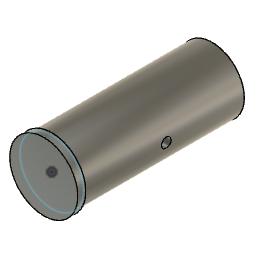
Small wrapped collar design _24 v3 (Autodesk Fusion 360 design; units mm, degrees)
Autodesk Fusion 360 part; units mm, degrees
sketch "Sketch2" plane through (0, 0, 0) normal (0, 0, 1) x (1, 0, 0)
  line L0 (0, 25.4) -> (10.16, 25.4)
  line L1 (0, 25.4) -> (0, 76.2)
  line L2 (10.16, 25.4) -> (10.16, 76.2)
  line L3 (10.16, 76.2) -> (0, 76.2)
  dimension "d47" = 10.16
  dimension "d48" = 50.8
  dimension "d49" = 50.8
  constraint horizontal L0
  constraint perpendicular L0 L1
  constraint perpendicular L0 L2
  measures "d47" distance of L0.start L0.end
  measures "d48" distance of L0.start L1.end
  measures "d49" distance of L0.end L2.end
revolve "Revolve1" add sketch "Sketch2" angle 360 about axis through (0, 25.4, 0) along (0, 1, 0) makes body 1
sketch "Sketch3" plane through (0, 76.2, 0) normal (0, 1, 0) x (-1, 0, 0)
  circle A0 centre (0, 0) radius 10.16
  circle A1 centre (0, 0) radius 5.08
  dimension "d6" = 10.16
  constraint coincident A0.centre A1.centre
  measures "d6" diameter of A1
sketch "Sketch7" plane through (0, 0, 0) normal (0, 0, 1) x (1, 0, 0)
  circle A0 through (2.5427, 49.9294, -10.5604) (-1.2073, 52.0944, -10.5604) (-1.2073, 47.7643, -10.5604)
  dimension "d15" = 5
sketch "Sketch8" plane through (0, 76.2, 0) normal (0, 1, 0) x (-1, 0, 0)
  circle A0 centre (0, 0) radius 10.16
  circle A1 centre (0, 0) radius 6.35
  dimension "d29" = 12.7
  constraint concentric A0 A1
  measures "d29" diameter of A1
hole "Hole4" at (-0.0344, 76.2, -0.1321) direction (0, -1, 0) diameter 15.3924 depth 50.8 tip angle 180 bodies 1
thread "Thread2" "ANSI Unified Screw Threads 0.6875 11/16-12 UN 2B" major diameter 17.4625 minor diameter 15.3924 pitch 2.1167 angle 60 resizes the face on face at (0.7319, 59.2667, 7.5258) on bodies 1
extrude "Extrude5" add sketch "Sketch3" against normal blind 50.8 separate body contours A1 makes body 2
hole "Hole5" at (-10.16, 51.5126, 0) direction (1, 0, 0) diameter 2.9972 depth 50.292 tip angle 118 bodies 1
move_face "OffsetFaces1" offset -38.1 1 faces at (1.2838, 76.2, 0.6601) on bodies 2
sketch "Sketch9" plane through (0, 25.4, 0) normal (0, -1, 0) x (1, 0, 0)
  circle A0 centre (0, 0) radius 5.08
  circle A1 centre (0, 0) radius 10.0907
  constraint coincident A0.centre A1.centre
sketch "Sketch10" plane through (0, 0, 0) normal (0, 1, 0) x (1, 0, 0)
  circle A0 centre (0, 0) radius 10.7615
  constraint coincident A0.centre origin
extrude "Extrude6" add sketch "Sketch10" along normal blind 2.54 separate body makes body 3
move_body "Move1" bodies 3 to x (1, 0, 0) y (0, 1, 0) z (0, 0, 1) at (0, 22.86, 0)
